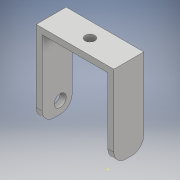
# Autodesk Inventor part: Hombro
Saved by Autodesk Inventor 2018 (Build 220112000, 112)
## iProperties
Created: 2020-03-07
Part Number: Hombro
Material: Generic
Document SubType Name: Modeling
Designer: GonzaloDiaz
Density: 1 g/cm^3
Appearance: Default
Mass: 41.36 g
Surface Area: 189.102 cm^2
Volume: 41.36 cm^3
Author: GonzaloDiaz
Autodesk Inventor part; units mm, degrees
ref_plane "YZ Plane" through (0, 0, 0) normal (1, 0, 0) x (0, 1, 0)
ref_plane "XZ Plane" through (0, 0, 0) normal (0, 1, 0) x (-1, 0, 0)
ref_plane "XY Plane" through (0, 0, 0) normal (0, 0, 1) x (1, 0, 0)
sketch "Sketch1" plane through (0, 0, 0) normal (0, 1, 0) x (-1, 0, 0)
  line L0 (0.1515, 5) -> (-4.8485, 5)
  line L1 (-4.8485, 5) -> (-4.8485, 75)
  line L2 (-4.8485, 75) -> (0.1515, 75)
  line L3 (0.1515, 75) -> (0.1515, 5)
  line L4 (54.9515, 5) -> (54.9515, 58.2)
  line L5 (54.9515, 5) -> (59.9515, 5)
  line L6 (59.9515, 5) -> (59.9515, 75)
  line L7 (59.9515, 75) -> (54.9515, 75)
  line L8 (54.9515, 75) -> (54.9515, 5)
  line L9 (0.1515, 75) -> (54.9515, 75)
  line L10 (54.9515, 75) -> (54.9515, 70)
  line L11 (54.9515, 70) -> (0.1515, 70)
  line L12 (0.1515, 70) -> (0.1515, 75)
  point P0 (0, 0)
  point P1 (55.2, 35)
  dimension "d0" = 5
  dimension "d1" = 70
  dimension "d2" = 5
  dimension "d3" = 5
  dimension "d10" = 54.8
  constraints: 26 end point, 6 parallel, 3 horizontal, 3 perpendicular, 2 point on line
  measures "d0" distance of L1.end L2.end
  measures "d1" distance of L0.end L1.end
  measures "d2" distance of L7.end L6.end
  measures "d3" distance of L9.end L10.end
  measures "d10" distance between parallel lines of L8 L3
extrude "Extrusion1" add sketch "Sketch1" along normal blind 25
fillet "Fillet1" radius 10 4 edges at (2.3485, 25, 5) (-57.4515, 25, 5) (2.3485, 0, 5) (-57.4515, 0, 5)
sketch "Sketch2" plane through (-59.9515, 0, 75) normal (-1, 0, 0) x (0, 0, 1)
  arc A0 (-60, 25) -> (-70, 15) centre (-60, 15) ccw projected
  circle A1 centre (-60, 15) radius 5
  point P0 (-75, 0)
  dimension "d7" = 10
  constraints: 1 centre point, 1 coincident
  measures "d7" diameter of A1
extrude "Extrusion2" cut sketch "Sketch2" against normal blind 5
sketch "Sketch3" plane through (-0.1515, 0, 70) normal (-1, 0, 0) x (0, 0, 1)
  circle A0 centre (-55, 15) radius 5 projected
  circle A1 centre (-55, 15) radius 5
  point P0 (-70, 0)
  constraints: 1 centre point, 1 coincident
sketch "Sketch4" plane through (-59.9515, 0, 75) normal (0, 0, 1) x (1, 0, 0)
  circle A0 centre (32.4, 12.5) radius 4
  line L0 (0, 0) -> (64.8, 0) projected
  line L1 (0, 0) -> (0, 25) projected
  point P0 (59.9515, 0)
  dimension "d11" = 8
  dimension "d12" = 12.5
  dimension "d13" = 32.4
  dimension "d14" = 25
  dimension "d15" = 64.8
  constraints: 1 centre point
  measures "d11" diameter of A0
  measures "d12" distance from line of L0 A0.centre
  measures "d13" distance from line of L1 A0.centre
  measures "d14" distance of L0.start L1.end
  measures "d15" distance of L0.start L0.end
extrude "Extrusion3" cut sketch "Sketch4" against normal blind 5
body "Solid1"
